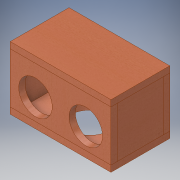
# Autodesk Inventor part: Front
Saved by Autodesk Inventor 2017 (Build 210142000, 142)
## iProperties
Created: 2019-01-31
Part Number: Front
Material: Generic
Document SubType Name: Modeling
Designer: Mitch
Density: 1 g/cm^3
Appearance: Walnut - Natural Polished
Author: Mitch
Autodesk Inventor part; units mm, degrees
ref_plane "YZ Plane" through (0, 0, 0) normal (1, 0, 0) x (0, 1, 0)
ref_plane "XZ Plane" through (0, 0, 0) normal (0, 1, 0) x (-1, 0, 0)
ref_plane "XY Plane" through (0, 0, 0) normal (0, 0, 1) x (1, 0, 0)
sketch "Sketch3" plane through (0, 0, 0) normal (0, 0, 1) x (1, 0, 0)
  line L0 (0, 0) -> (304.8, 0)
  line L1 (304.8, 0) -> (304.8, 152.4)
  line L2 (304.8, 152.4) -> (0, 152.4)
  line L3 (0, 152.4) -> (0, 0)
  dimension "d12" = 304.8
  dimension "d13" = 152.4
  constraints: 8 end point, 2 parallel, 1 horizontal, 1 perpendicular
  measures "d12" distance of L2.end L1.end
  measures "d13" distance of L1.end L0.end
extrude "Extrusion3" add sketch "Sketch3" along normal blind 19.05
sketch "Sketch4" plane through (0, 0, 19.05) normal (0, 0, 1) x (1, 0, 0)
  circle A0 centre (76.2, 63.5) radius 50.8
  circle A1 centre (228.6, 63.5) radius 50.8
  line L0 (0, 152.4) -> (0, 0) projected
  line L1 (304.8, 152.4) -> (0, 152.4) projected
  line L2 (304.8, 0) -> (304.8, 152.4) projected
  dimension "d16" = 101.6
  dimension "d17" = 101.6
  dimension "d18" = 76.2
  dimension "d19" = 88.9
  dimension "d20" = 88.9
  dimension "d21" = 76.2
  constraints: 2 centre point
  measures "d16" diameter of A0
  measures "d17" diameter of A1
  measures "d18" distance from line of L0 A0.centre
  measures "d19" distance from line of L1 A0.centre
  measures "d20" distance from line of L1 A1.centre
  measures "d21" distance from line of L2 A1.centre
extrude "Extrusion4" cut sketch "Sketch4" against normal blind 25.4
sketch "Sketch5" plane through (0, 152.4, 0) normal (0, 1, 0) x (1, 0, 0)
  line L0 (304.8, -19.05) -> (0, -19.05) projected
  line L1 (304.8, -19.05) -> (0, -19.05)
  line L2 (0, -19.05) -> (0, 158.75)
  line L3 (0, 158.75) -> (304.8, 158.75)
  line L4 (304.8, 158.75) -> (304.8, -19.05)
  point P0 (0, 0)
  dimension "d24" = 177.8
  constraints: 8 end point, 2 parallel, 1 horizontal, 1 perpendicular
  measures "d24" distance of L3.end L0.start
extrude "Extrusion5" add sketch "Sketch5" along normal blind 19.05 separate body
sketch "Sketch6" plane through (0, 0, 0) normal (0, -1, 0) x (1, 0, 0)
  line L0 (0, -158.75) -> (0, 19.05) projected
  line L1 (304.8, 19.05) -> (304.8, -158.75) projected
  line L2 (0, 19.05) -> (304.8, 19.05)
  line L3 (304.8, 19.05) -> (304.8, -158.75)
  line L4 (304.8, -158.75) -> (0, -158.75)
  line L5 (0, -158.75) -> (0, 19.05)
  point P0 (0, 0)
  constraints: 8 end point, 2 parallel, 1 horizontal, 1 perpendicular
extrude "Extrusion6" add sketch "Sketch6" along normal blind 19.05 separate body
sketch "Sketch7" plane through (0, -19.05, 0) normal (0, -1, 0) x (1, 0, 0)
  circle A0 centre (152.4, -69.85) radius 60.325
  line L0 (0, 19.05) -> (0, -158.75) projected
  line L1 (304.8, -158.75) -> (0, -158.75) projected
  point P0 (0, 0)
  dimension "d29" = 120.65
  dimension "d30" = 152.4
  dimension "d31" = 88.9
  constraints: 1 centre point
  measures "d29" diameter of A0
  measures "d30" distance from line of L0 A0.centre
  measures "d31" distance from line of L1 A0.centre
extrude "Extrusion7" cut sketch "Sketch7" against normal blind 25.4 bodies 3
sketch "Sketch8" plane through (0, 0, 0) normal (0, 0, -1) x (-1, 0, 0)
  line L0 (-304.8, 152.4) -> (0, 152.4) projected
  line L1 (0, 0) -> (-304.8, 0) projected
  line L2 (0, 152.4) -> (-19.05, 152.4)
  line L3 (-19.05, 152.4) -> (-19.05, 0)
  line L4 (-19.05, 0) -> (0, 0)
  line L5 (0, 0) -> (0, 152.4)
  dimension "d34" = 19.05
  constraints: 8 end point, 2 parallel, 1 horizontal, 1 perpendicular, 1 point on line
  measures "d34" distance between parallel lines of L5 L3
extrude "Extrusion8" add sketch "Sketch8" along normal blind 139.7 separate body
sketch "Sketch9" plane through (0, 0, 0) normal (0, 0, -1) x (-1, 0, 0)
  line L0 (0, 0) -> (-304.8, 0) projected
  line L1 (-304.8, 152.4) -> (-285.75, 152.4)
  line L2 (-285.75, 152.4) -> (-285.75, 0)
  line L3 (-285.75, 0) -> (-304.8, 0)
  line L4 (-304.8, 0) -> (-304.8, 152.4)
  dimension "d37" = 19.05
  constraints: 8 end point, 2 parallel, 1 horizontal, 1 perpendicular, 1 point on line
  measures "d37" distance between parallel lines of L4 L2
extrude "Extrusion9" add sketch "Sketch9" along normal blind 139.7 separate body
sketch "Sketch10" plane through (0, 0, -139.7) normal (0, 0, -1) x (-1, 0, 0)
  line L0 (-285.75, 152.4) -> (-304.8, 152.4) projected
  line L1 (-304.8, 152.4) -> (0, 152.4)
  line L2 (0, 152.4) -> (0, 0)
  line L3 (0, 0) -> (-304.8, 0)
  line L4 (-304.8, 0) -> (-304.8, 152.4)
  constraints: 8 end point, 2 parallel, 1 horizontal, 1 perpendicular
extrude "Extrusion10" add sketch "Sketch10" along normal blind 19.05 separate body
